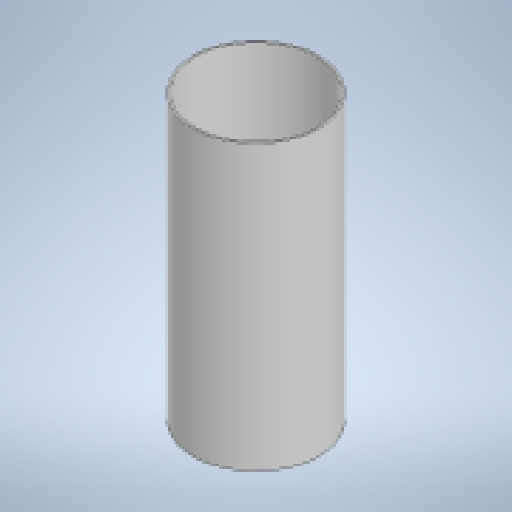
# Autodesk Inventor part: ДМФ 056 труба илоотвода v2.1
Saved by Autodesk Inventor 2026.2 (Build 302298000, 298)
## iProperties
Created: 2024-05-13
Part Number: ДМФ 056 труба илоотвода v2.1
Material: Generic
Document SubType Name: Modeling
Designer: admin
Density: 1 g/cm^3
Appearance: Default
Author: admin
Autodesk Inventor part; units mm, degrees
ref_plane "YZ Plane" through (0, 0, 0) normal (1, 0, 0) x (0, 1, 0)
ref_plane "XZ Plane" through (0, 0, 0) normal (0, 1, 0) x (-1, 0, 0)
ref_plane "XY Plane" through (0, 0, 0) normal (0, 0, 1) x (1, 0, 0)
sketch "Sketch1" plane through (0, 0, 0) normal (0, 0, 1) x (1, 0, 0)
  circle A0 centre (0, 0) radius 66.5
  circle A1 centre (0, 0) radius 61.5
  dimension "d0" = 133
  dimension "d1" = 5
  constraints: 2 centre point, 1 coincident
  measures "d0" diameter of A0
  measures "d1" radial gap between concentric circles of A0 A1
extrude "Extrusion1" add sketch "Sketch1" along normal blind 300 contours A0 | A1
shell "Shell1" thickness 2 removed faces 2 at (16.5265, 16.6399, 300) at (16.5265, 16.6399, 0)
body "Solid1"
